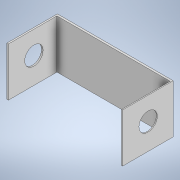
# Autodesk Inventor part: clamp 2
Saved by Autodesk Inventor 2020 (Build 240168000, 168)
## iProperties
Created: 2020-02-18
Part Number: clamp 2
Material: Generic
Document SubType Name: Modeling
Designer: Hp
Density: 1 g/cm^3
Appearance: Default
Author: Hp
Autodesk Inventor part; units mm, degrees
ref_plane "YZ Plane" through (0, 0, 0) normal (1, 0, 0) x (0, 1, 0)
ref_plane "XZ Plane" through (0, 0, 0) normal (0, 1, 0) x (-1, 0, 0)
ref_plane "XY Plane" through (0, 0, 0) normal (0, 0, 1) x (1, 0, 0)
sketch "Sketch1" plane through (0, 0, 0) normal (1, 0, 0) x (0, 1, 0)
  line L0 (1.8986, 1.3831) -> (-40.1014, 1.3831)
  line L1 (-40.1014, 1.3831) -> (-40.1014, -42.3731)
  line L2 (-40.1014, -42.3731) -> (1.8986, -42.3731)
  line L3 (1.8986, -42.3731) -> (1.8986, 1.3831)
  point P0 (0, 0)
  dimension "d0" = 42
  constraints: 8 end point, 2 parallel, 1 horizontal, 1 perpendicular
  measures "d0" distance of L2.end L1.end
extrude "Extrusion1" add sketch "Sketch1" along normal blind 100
sketch "Sketch3" plane through (0, 0, 0) normal (-1, 0, 0) x (0, 0, 1)
  point P0 (0, 0)
sketch "Sketch8" plane through (0, 0, 0) normal (-1, 0, 0) x (0, 0, 1)
  point P0 (0, 0)
  point P1 (-20.6894, -17.7504)
hole "Hole4" at (0, -17.7504, -20.6894) direction (1, 0, 0) diameter 15.875 end through all
sketch "Sketch9" plane through (0, -40.1014, 1.3831) normal (0, 0, 1) x (1, 0, 0)
  line L0 (0, 42) -> (100, 42) projected
  line L1 (0, 0) -> (100, 0) projected
  line L2 (1.351, 42) -> (99.1356, 42)
  line L3 (99.1356, 42) -> (99.1356, 0)
  line L4 (99.1356, 0) -> (1.351, 0)
  line L5 (1.351, 0) -> (1.351, 42)
  point P0 (0, 40.1014)
  point P1 (1.351, 0)
  constraints: 8 end point, 2 parallel, 2 point on line, 1 horizontal, 1 perpendicular
extrude "Extrusion4" cut sketch "Sketch9" against normal blind 42
body "Solid1"
